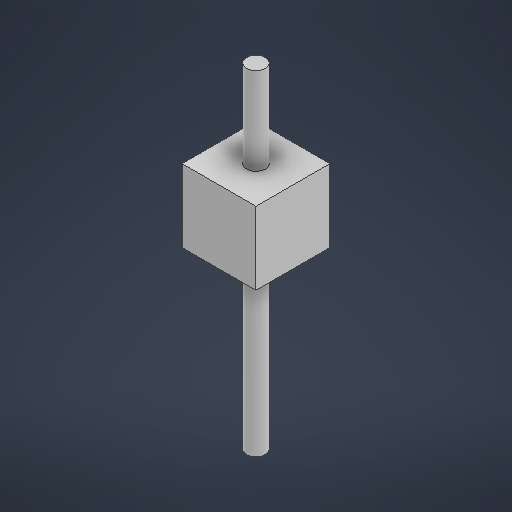
# Autodesk Inventor part: pin-header-male
Saved by Autodesk Inventor 2025.2 (Build 292293000, 293)
## iProperties
Created: 2025-11-15
Part Number: pin-header-male
Material: Aluminum
Document SubType Name: Modeling
Designer: sam
Density: 2.7 g/cm^3
Appearance: Satin - Silver
Author: sam
Autodesk Inventor part; units mm, degrees
ref_plane "YZ Plane" through (0, 0, 0) normal (1, 0, 0) x (0, 1, 0)
ref_plane "XZ Plane" through (0, 0, 0) normal (0, 1, 0) x (-1, 0, 0)
ref_plane "XY Plane" through (0, 0, 0) normal (0, 0, 1) x (1, 0, 0)
sketch "Sketch1" plane through (0, 0, 0) normal (0, 1, 0) x (-1, 0, 0)
  line L0 (-1.27, -1.27) -> (1.27, -1.27)
  line L1 (1.27, -1.27) -> (1.27, 1.27)
  line L2 (1.27, 1.27) -> (-1.27, 1.27)
  line L3 (-1.27, 1.27) -> (-1.27, -1.27)
  line L4 (-1.27, -1.27) -> (1.27, 1.27) construction
  line L5 (1.27, -1.27) -> (-1.27, 1.27) construction
  point P0 (0, 0)
  dimension "d0" = 2.54
  dimension "d1" = 2.54
  constraints: 12 end point, 2 midpoint, 2 parallel, 1 horizontal, 1 perpendicular
  measures "d0" distance of L2.end L1.end
  measures "d1" distance of L1.end L0.end
extrude "Extrusion1" add sketch "Sketch1" along normal blind 2.5
sketch "Sketch2" plane through (0, 2.5, 0) normal (0, 1, 0) x (1, 0, 0)
  circle A0 centre (0, 0) radius 0.325
  dimension "d4" = 0.65
  constraints: 1 centre point, 1 coincident
  measures "d4" diameter of A0
extrude "Extrusion2" add sketch "Sketch2" along normal blind 3
sketch "Sketch3" plane through (0, 0, 0) normal (0, -1, 0) x (1, 0, 0)
  circle A0 centre (0, 0) radius 0.325
  dimension "d7" = 0.65
  constraints: 1 centre point, 1 coincident
  measures "d7" diameter of A0
extrude "Extrusion3" add sketch "Sketch3" along normal blind 6
body "Solid1"
